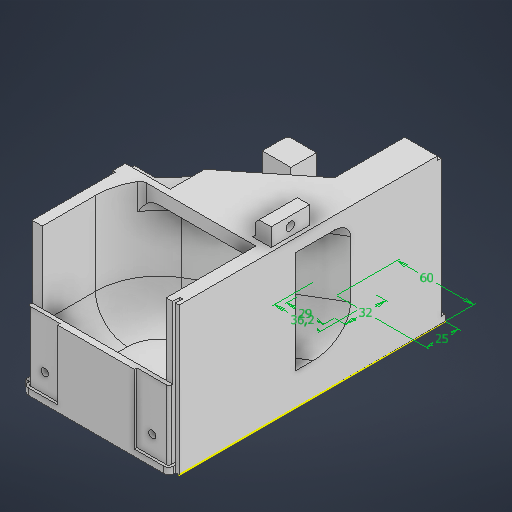
# Autodesk Inventor part: Rampe_V2
Saved by Autodesk Inventor 2026.1 (Build 301233020, 233B)
## iProperties
Created: 2025-05-14
Part Number: Rampe_V2
Material: Generisch
Document SubType Name: Modeling
Designer: iopeter
Density: 1 g/cm^3
Appearance: Vorgabe
Author: iopeter
Autodesk Inventor part; units mm, degrees
ref_plane "YZ Plane" through (0, 0, 0) normal (1, 0, 0) x (0, 1, 0)
ref_plane "XZ Plane" through (0, 0, 0) normal (0, 1, 0) x (-1, 0, 0)
ref_plane "XY Plane" through (0, 0, 0) normal (0, 0, 1) x (1, 0, 0)
ref_plane "Arbeitsebene1" through (-48.5, 0, 84.5) normal (1, 0, 0) x (0, 0, -1)
sketch "Skizze1" plane through (-48.5, 0, 84.5) normal (1, 0, 0) x (0, 0, -1)
  line L0 (81.5, 430) -> (81.5, -250) construction
  line L1 (-117.5, 430) -> (81.5, 430) construction
  line L2 (-117.5, -250) -> (-117.5, 430) construction
  line L3 (81.5, -250) -> (-117.5, -250) construction
  line L4 (81.5, -360) -> (-117.5, -360) construction
  line L5 (-117.5, -360) -> (-117.5, 430) construction
  line L6 (84.5, -360) -> (84.5, 430) construction
  line L7 (84.5, -360) -> (-117.5, -360)
  line L8 (-117.5, -360) -> (-117.5, -250)
  line L9 (-117.5, -250) -> (84.5, -250)
  line L10 (84.5, -250) -> (84.5, -360)
  line L11 (-117.5, -250) -> (-47.5, -250)
  line L12 (-47.5, -250) -> (-47.5, -340)
  line L13 (-47.5, -340) -> (-117.5, -340)
  line L14 (-117.5, -340) -> (-117.5, -250)
  point P0 (84.5, 0)
  point P1 (-117.5, -340)
  dimension "d7" = 70
  dimension "d8" = 90
  constraints: 16 end point, 4 parallel, 2 horizontal, 2 perpendicular, 1 point on line
  measures "d7" distance of L12.end L13.end
  measures "d8" distance of L11.end L12.end
ref_plane "Arbeitsebene2" through (68.5, -430, -3) normal (1, 0, 0) x (0, 1, 0)
extrude "Extrusion1" add sketch "Skizze1" along normal up to surface (117 mm away)
ref_plane "Arbeitsebene4" through (-38.5, 0, 84.5) normal (-1, 0, 0) x (0, 0, 1)
sketch "Skizze4" plane through (-38.5, 0, 84.5) normal (-1, 0, 0) x (0, 0, 1)
  line L0 (47.5, -340) -> (117.5, -340) projected
  line L1 (47.5, -250) -> (47.5, -340) projected
  line L2 (117.5, -250) -> (117.5, -360) projected
  line L3 (-84.5, -360) -> (-84.5, -250) projected
  line L4 (117.5, -360) -> (-84.5, -360) projected
  line L5 (117.5, -250) -> (117.5, -360) projected
  line L6 (-84.5, -250) -> (117.5, -250) projected
  point P0 (-84.5, 0)
extrude "Extrusion4" cut sketch "Skizze4" against normal through all contours L1 L6 L2 L0
sketch "Skizze5" plane through (-38.5, -340, 202) normal (0, 1, 0) x (1, 0, 0)
  line L0 (0, 70) -> (107, 70) projected
  line L1 (107, 70) -> (107, 202) projected
  line L2 (-10, 202) -> (107, 202) projected
  line L3 (-10, 202) -> (-10, 0) projected
  line L4 (-10, 0) -> (0, 0) projected
  line L5 (0, 0) -> (0, 70) projected
  line L6 (0, 70) -> (107, 134)
  point P0 (38.5, 202)
  dimension "d17" = 68
  constraints: 2 end point, 1 point on line
  measures "d17" distance of L1.end L6.end
extrude "Extrusion5" cut sketch "Skizze5" along normal blind 80 contours L6 L1 L0
fillet "Rundung1" radius 50 1 edges at (-38.5, -300, 132)
fillet "Rundung2" radius 25 4 edges at (-31.993, -340, 135.6901) (-38.5, -340, 171.1775) (-38.5, -340, 192) (27.1671, -340, 92.7225)
fillet "Rundung3" radius 10.5 2 edges at (-22.7072, -260, 123.8876) (27.1671, -260, 92.7225)
fillet "Rundung5" radius 3.5 1 edges at (-48.5, -305, 0)
fillet "Rundung8" radius 5 2 edges at (-29.6825, -265.25, 132) (-29.6825, -255, 132)
sketch "Skizze10" plane through (68.5, -340, 202) normal (1, 0, 0) x (0, 0, -1)
  line L0 (70, 90) -> (202, 90) projected
  line L1 (202, 90) -> (202, -20) projected
  line L2 (0, -20) -> (0, 0) projected
  line L3 (0, 0) -> (104.8693, 0) projected
  ellipse E0 centre (104.8693, 25) end of major axis (134, 25) minor radius 25 (104.8693, 0) -> (134, 25) ccw projected
  line L4 (134, 25) -> (134, 69.5) projected
  ellipse E1 centre (121.7651, 69.5) end of major axis (134, 69.5) minor radius 10.5 (134, 69.5) -> (121.7651, 80) ccw projected
  line L5 (121.7651, 80) -> (70, 80) projected
  line L6 (0, 0) -> (71, 0)
  line L7 (71, 0) -> (71, 90)
  line L8 (71, 90) -> (0, 90)
  line L9 (0, 90) -> (0, 0)
  line L10 (70, 80) -> (70, 90) projected
  line L11 (202, -20) -> (0, -20) projected
  point P0 (202, 340)
  point P1 (71, 80)
  constraints: 8 end point, 2 parallel, 1 horizontal, 1 perpendicular, 2 other
extrude "Extrusion9" add sketch "Skizze10" against normal blind 10 contours L10 L5 L7 L3 L9 L8
thicken "Thicken2" operation add thickness 20 both sides no extend neighbours no toward (0, 0, -1) faces at (61.8333, -313.3333, 131)
sketch "Sketch13" plane through (-48.5, -360, 202) normal (0, -1, 0) x (1, 0, 0)
  arc A0 (0, -198.5) -> (3.5, -202) centre (3.5, -198.5) ccw projected
  line L0 (3.5, -202) -> (117, -202) projected
  line L1 (117, -202) -> (117, 0) projected
  line L2 (0, 0) -> (117, 0) projected
  line L3 (0, 0) -> (0, -198.5) projected
  line L4 (-3, -199) -> (0, -199) projected
  line L5 (0, -199) -> (0, 0) projected
  line L6 (-3, 0) -> (0, 0) projected
  line L7 (-3, 0) -> (-3, -199) projected
  line L8 (3, -205) -> (3, -202) projected
  arc A1 (0, -199) -> (3, -202) centre (3, -199) ccw projected
  line L9 (-3, -199) -> (0, -199) projected
  arc A2 (-3, -199) -> (3, -205) centre (3, -199) ccw projected
  line L10 (111, -205) -> (111, -202) projected
  line L11 (111, -202) -> (3, -202) projected
  line L12 (3, -205) -> (3, -202) projected
  line L13 (3, -205) -> (111, -205) projected
  line L14 (117, -202) -> (111, -202)
  line L15 (111, -202) -> (111, -205)
  line L16 (111, -205) -> (117, -205)
  line L17 (117, -205) -> (117, -202)
  point P0 (48.5, -202)
  constraints: 8 end point, 2 parallel, 1 horizontal, 1 perpendicular
extrude "Extrusion11" add sketch "Sketch13" along normal blind 5
fillet "Fillet10" radius 2 1 edges at (68.5, -362.5, -3)
sketch "Sketch14" plane through (-48.5, -365, 202) normal (0, -1, 0) x (1, 0, 0)
  line L0 (27, 5) -> (4, 5) projected
  arc A0 (4, 5) -> (0, 1) centre (4, 1) ccw projected
  line L1 (0, 1) -> (0, -65) projected
  line L2 (110, 5) -> (87, 5) projected
  arc A1 (114, 1) -> (110, 5) centre (110, 1) ccw projected
  line L3 (114, -65) -> (114, 1) projected
  line L4 (27, 5) -> (87, 5)
  line L5 (0, 0) -> (10, 0) projected
  line L6 (0, 0) -> (114, 0)
  point P0 (48.5, -202)
  constraints: 4 end point, 1 collinear, 1 perpendicular, 1 point on line
ref_plane "Work Plane5" through (38.5, -360, 205) normal (0, -1, 0) x (1, 0, 0)
extrude "Extrusion12" add sketch "Sketch14" against normal up to surface (5 mm away)
sketch "Sketch15" plane through (-48.5, -360, 202) normal (0, 1, 0) x (1, 0, 0)
  line L0 (4, -3) -> (27, -3)
  arc A0 (2, -1) -> (4, -3) centre (4, -1) ccw
  line L1 (2, 65) -> (2, -1)
  line L2 (87, -3) -> (110, -3)
  arc A1 (110, -3) -> (112, -1) centre (110, -1) ccw
  line L3 (112, -1) -> (112, 65)
  line L4 (27, -3) -> (87, -3)
  line L5 (107, 0) -> (35, 0)
  line L6 (2, -1) -> (2, 0)
  line L7 (2, 0) -> (112, 0)
  line L8 (112, 0) -> (112, -1)
  arc A2 (110, -3) -> (112, -1) centre (110, -1) ccw
  line L9 (110, -3) -> (87, -3)
  line L10 (87, -3) -> (87, -5)
  line L11 (87, -5) -> (27, -5)
  line L12 (27, -3) -> (27, -5)
  line L13 (27, -3) -> (4, -3)
  arc A3 (2, -1) -> (4, -3) centre (4, -1) ccw
  point P0 (48.5, 202)
extrude "Extrusion13" add sketch "Sketch15" along normal blind 54 contours A0 L1 L7 L5 L3 A1 L2 L4 L0
sketch "Sketch16" plane through (-44.5, -360, 205) normal (0, 0, 1) x (1, 0, 0)
  line L0 (0, 790) -> (0, 0) projected
  line L1 (23, 0) -> (0, 0) projected
  line L2 (23, 117) -> (23, 0) projected
  line L3 (27.5, 117) -> (23, 117) projected
  line L4 (27.5, 674) -> (27.5, 117) projected
  line L5 (23, 674) -> (27.5, 674) projected
  line L6 (23, 790) -> (23, 674) projected
  line L7 (0, 790) -> (23, 790) projected
  line L8 (106, 0) -> (106, 790) projected
  line L9 (83, 790) -> (106, 790) projected
  line L10 (83, 674) -> (83, 790) projected
  line L11 (78.5, 674) -> (83, 674) projected
  line L12 (78.5, 117) -> (78.5, 674) projected
  line L13 (83, 117) -> (78.5, 117) projected
  line L14 (83, 0) -> (83, 117) projected
  line L15 (106, 0) -> (83, 0) projected
  line L16 (106, 0) -> (0, 0) projected
  line L17 (106, 0) -> (106, 54) projected
  line L18 (0, 54) -> (106, 54) projected
  line L19 (0, 0) -> (0, 54) projected
  point P0 (44.5, 360)
  point P1 (83, 54)
  point P2 (23, 54)
ref_plane "Work Plane6" through (-44.5, -360, 207) normal (0, 0, 1) x (1, 0, 0)
extrude "Extrusion14" add sketch "Sketch16" along normal up to surface (2 mm away) contours L18 L14 L16 L2
sketch "Sketch17" plane through (-48.5, -360, 202) normal (0, 1, 0) x (1, 0, 0)
  line L0 (111, 205) -> (111, 202) construction
  arc A0 (117, 203) -> (115, 205) centre (115, 203) ccw construction
  line L1 (3, 205) -> (115, 205) construction
  arc A1 (3, 205) -> (-3, 199) centre (3, 199) ccw projected
  line L2 (-3, 0) -> (-3, 199) projected
  line L3 (0, 0) -> (-3, 0) projected
  line L4 (0, 0) -> (0, 198.5) projected
  arc A2 (3.5, 202) -> (0, 198.5) centre (3.5, 198.5) ccw projected
  line L5 (3.5, 202) -> (117, 202) construction
  line L6 (117, 203) -> (117, 202) construction
  line L7 (111, 202) -> (117, 202)
  line L8 (117, 202) -> (117, 205)
  line L9 (117, 205) -> (111, 205)
  line L10 (111, 205) -> (111, 202)
  point P0 (48.5, 202)
  constraints: 8 end point, 2 parallel, 1 horizontal, 1 perpendicular, 1 other
extrude "Extrusion15" add sketch "Sketch17" along normal blind 107 and the other way blind 5
sketch "Sketch18" plane through (-48.5, -365, 202) normal (0, -1, 0) x (1, 0, 0)
  line L0 (3, -208) -> (117, -208) projected
  line L1 (117, -205) -> (117, -208) projected
  line L2 (117, -205) -> (3, -205) projected
  line L3 (3, -205) -> (3, -208) projected
  point P0 (48.5, -202)
ref_plane "Work Plane7" through (-45.5, -360, -6) normal (0, -1, 0) x (1, 0, 0)
extrude "Extrusion16" add sketch "Sketch18" against normal up to surface (5 mm away)
sketch "Sketch19" plane through (-48.5, 0, 84.5) normal (-1, 0, 0) x (0, 0, 1)
  line L0 (48.5, 430) -> (48.5, -360) projected
  circle A0 centre (108.5, 160) radius 2.5 projected
  circle A1 centre (108.5, -135) radius 2.5 projected
  line L1 (52.5, 430) -> (52.5, -360) projected
  line L2 (118.5, -360) -> (52.5, -360) projected
  line L3 (118.5, 430) -> (118.5, -360) projected
  line L4 (52.5, 430) -> (118.5, 430) projected
  line L5 (48.5, -360) -> (118.5, -360)
  line L6 (118.5, -360) -> (118.5, -250)
  line L7 (118.5, -250) -> (48.5, -250)
  line L8 (48.5, -250) -> (48.5, -360)
  point P0 (-84.5, 0)
  point P1 (117.5, -250)
  point P2 (48.5, -250)
  point P3 (52.5, -250)
  constraints: 8 end point, 2 parallel, 1 horizontal, 1 horizontal alignment, 1 perpendicular, 1 point on line
extrude "Extrusion17" cut sketch "Sketch19" against normal blind 2 contours L7 L3 L2 L1
sketch "Sketch21" plane through (68.5, -250, 202) normal (0, 1, 0) x (1, 0, 0)
  line L0 (0, 0) -> (0, 202) projected
  line L1 (0, 75) -> (-15, 75)
  line L2 (-15, 75) -> (-15, 105)
  line L3 (-15, 105) -> (0, 105)
  line L4 (0, 105) -> (0, 75)
  line L5 (0, 75) -> (-3, 75)
  line L6 (-3, 75) -> (-3, 105)
  line L7 (-3, 105) -> (0, 105)
  line L8 (0, 105) -> (0, 75)
  point P0 (-68.5, 202)
  point P1 (0, 105)
  point P2 (-3, 75)
  dimension "d131" = 15
  dimension "d132" = 30
  dimension "d133" = 75
  dimension "d143" = 3
  constraints: 16 end point, 4 parallel, 2 horizontal, 2 perpendicular, 2 point on line
  measures "d131" distance of L2.end L3.end
  measures "d132" distance of L1.end L2.end
  measures "d133" distance of L0.start L1.start
  measures "d143" distance of L6.end L7.end
extrude "Extrusion19" add sketch "Sketch21" along normal blind 14 contours L1 L2 L3 L6
sketch "Sketch22" plane through (-38.5, -250, 202) normal (0, 1, 0) x (1, 0, 0)
  line L0 (102, 5) -> (104, 5) projected
  line L1 (104, 5) -> (104, -1) projected
  line L2 (102, -1) -> (104, -1) projected
  line L3 (102, -1) -> (102, 5) projected
  line L4 (102, -1) -> (104, -1) projected
  arc A0 (100, -5) -> (104, -1) centre (100, -1) ccw projected
  line L5 (100, -3) -> (100, -5) projected
  arc A1 (100, -3) -> (102, -1) centre (100, -1) ccw projected
  point P0 (38.5, 202)
extrude "Extrusion20" cut sketch "Sketch22" against normal up to surface (110 mm away) contours L0 L1 L2 L3
thicken "Thicken3" operation cut thickness 0.5 both sides no extend neighbours no toward (0, 0, -1) faces at (64.8333, -323.3333, 197)
sketch "Sketch24" plane through (65.5, -250, 127) normal (1, 0, 0) x (0, 0, -1)
  line L0 (30, 0) -> (0, 0) projected
  line L1 (30, 0) -> (30, 14) projected
  line L2 (0, 14) -> (30, 14) projected
  line L3 (0, 0) -> (0, 14) projected
  circle A0 centre (15, 7) radius 3.2
  point P0 (127, 250)
  point P1 (0, 7)
  point P2 (15, 14)
  dimension "d144" = 6.4
  constraints: 2 midpoint, 1 centre point, 1 horizontal alignment, 1 vertical alignment
  measures "d144" diameter of A0
extrude "Extrusion22" cut sketch "Sketch24" against normal through all contours A0
chamfer "Chamfer15" distance 2.5 angle 45 1 edges at (53.5, -250, 112)
chamfer "Chamfer16" distance 2.5 angle 45 1 edges at (53.5, -236, 112)
sketch "Sketch25" plane through (-44.5, -360, 205) normal (0, 0, 1) x (1, 0, 0)
  circle A0 centre (11, 775) radius 2.8 projected
  circle A1 centre (95, 775) radius 2.8 projected
  circle A2 centre (95, 15) radius 2.8
  circle A3 centre (11, 15) radius 2.8
  line L0 (23, 0) -> (0, 0) projected
  point P0 (44.5, 360)
  dimension "d153" = 15
  constraints: 2 centre point, 2 equal radius, 2 vertical alignment, 1 horizontal alignment
  measures "d153" distance from line of L0 A3.centre
extrude "Extrusion23" cut sketch "Sketch25" against normal blind 12 contours A2 | A3
sketch "Skizze26" plane through (-48.5, 0, 84.5) normal (-1, 0, 0) x (0, 0, 1)
  line L0 (12.5, -250) -> (42.5, -250) projected
  line L1 (42.5, -250) -> (-70.5, -250)
  line L2 (-70.5, -250) -> (-70.5, -255)
  line L3 (-70.5, -255) -> (42.5, -255)
  line L4 (42.5, -255) -> (42.5, -250)
  circle A0 centre (18.5, -229.9838) radius 11 projected
  circle A1 centre (-46.5, -229.9838) radius 11 projected
  point P0 (-84.5, 0)
  dimension "d156" = 5
  dimension "d157" = 24
  constraints: 8 end point, 2 parallel, 1 horizontal, 1 perpendicular
  measures "d156" distance between parallel lines of L3 L1
  measures "d157" distance from line of L2 A1.centre
extrude "Extrusion24" cut sketch "Skizze26" against normal blind 35 contours L0 L4 L3 L2 L1
sketch "Skizze27" plane through (-48.5, -365, 202) normal (0, -1, 0) x (1, 0, 0)
  line L0 (42.5, -199) -> (71.5, -199)
  line L1 (71.5, -199) -> (71.5, -167)
  line L2 (71.5, -167) -> (42.5, -167)
  line L3 (42.5, -167) -> (42.5, -199)
  line L4 (42.5, -199) -> (71.5, -167) construction
  line L5 (71.5, -199) -> (42.5, -167) construction
  line L6 (38.9, -183) -> (75.1, -183) construction
  line L7 (117, -208) -> (117, 0) projected
  line L8 (3, -208) -> (117, -208) projected
  point P0 (48.5, -202)
  point P1 (57, -183)
  point P2 (57, -183)
  dimension "d162" = 29
  dimension "d163" = 32
  dimension "d164" = 36.2
  dimension "d165" = 60
  dimension "d166" = 25
  constraints: 14 end point, 3 midpoint, 2 coincident, 2 horizontal, 2 parallel, 1 perpendicular
  measures "d162" distance of L2.end L1.end
  measures "d163" distance of L1.end L0.end
  measures "d164" distance of L6.end L6.start
  measures "d165" distance from line of point (57, -183) L7
  measures "d166" distance from line of L8 point (57, -183)
extrude "Extrusion25" cut sketch "Skizze27" against normal blind 120.75
hole "Bohrung3" at (-9.6, -365, 19) at (26.6, -365, 19) direction (0, 1, 0) diameter 3.3 end through all
thicken "Thicken4" operation cut thickness 0.1 both sides no extend neighbours no toward (1, 0, 0) faces at (65.5, -286.6667, 200.1667)
sketch "Sketch28" plane through (68.5, -250, 202) normal (0, 1, 0) x (1, 0, 0)
  line L0 (-113.5, 202) -> (-6, 202) projected
  line L1 (-25.5, 202) -> (-94.5, 202)
  line L2 (-94.5, 202) -> (-94.5, 147)
  line L3 (-94.5, 147) -> (-25.5, 147)
  line L4 (-25.5, 147) -> (-25.5, 202)
  line L5 (-45.5, 199) -> (-45.5, 167) projected
  line L6 (-74.5, 167) -> (-74.5, 199) projected
  line L7 (-45.5, 167) -> (-74.5, 167) projected
  point P0 (-68.5, 202)
  dimension "d178" = 20
  dimension "d179" = 20
  dimension "d180" = 20
  constraints: 8 end point, 2 parallel, 1 horizontal, 1 perpendicular, 1 point on line
  measures "d178" distance between parallel lines of L4 L5
  measures "d179" distance between parallel lines of L6 L2
  measures "d180" distance between parallel lines of L7 L3
extrude "Extrusion26" cut sketch "Sketch28" against normal blind 100
sketch "Sketch29" plane through (-45, -360, 0) normal (0, 0, -1) x (-1, 0, 0)
  circle A0 centre (-101.5, 55.0162) radius 3 construction
  circle A1 centre (-11.5, 55.0162) radius 3 construction
  circle A2 centre (-101.5, 55.0162) radius 3.2
  circle A3 centre (-11.5, 55.0162) radius 3.2
  point P0 (-45, 360)
  dimension "d183" = 6.4
  dimension "d184" = 6.4
  constraints: 4 coincident, 2 centre point
  measures "d183" diameter of A2
  measures "d184" diameter of A3
extrude "Extrusion27" cut sketch "Sketch29" against normal blind 15
sketch "Skizze30" plane through (68.5, -250, 202) normal (0, 1, 0) x (1, 0, 0)
  line L0 (0, 134) -> (-82.6658, 84.555) projected
  line L1 (-82, 75) -> (-82, 147) projected
  line L2 (-117, 202) -> (-82, 202)
  line L3 (-82, 202) -> (-82, 102)
  line L4 (-82, 102) -> (-117, 102)
  line L5 (-117, 102) -> (-117, 202)
  line L6 (-25.5, 147) -> (-82, 147) projected
  line L7 (-82, 102) -> (-25.5, 147)
  point P0 (-68.5, 202)
  point P1 (-113.5, 202)
  point P2 (-117, 198.5)
  dimension "d187" = 100
  constraints: 10 end point, 2 parallel, 1 horizontal, 1 horizontal alignment, 1 perpendicular, 1 point on line, 1 vertical alignment
  measures "d187" distance of L2.end L3.end
extrude "Extrusion28" cut sketch "Skizze30" against normal blind 45
sketch "Skizze31" plane through (68.5, -295, 202) normal (0, 1, 0) x (1, 0, 0)
  line L0 (-94.5, 147) -> (-25.5, 147) projected
  line L1 (-94.5, 202) -> (-94.5, 147) projected
  line L2 (-113.5, 202) -> (-94.5, 202) projected
  arc A0 (-113.5, 202) -> (-117, 198.5) centre (-113.5, 198.5) ccw projected
  line L3 (-117, 102) -> (-117, 198.5) projected
  line L4 (-82, 102) -> (-117, 102) projected
  line L5 (-25.5, 147) -> (-82, 102) projected
  line L6 (-94.5, 202) -> (-117, 202)
  line L7 (-117, 202) -> (-117, 182)
  line L8 (-117, 182) -> (-94.5, 182)
  line L9 (-94.5, 182) -> (-94.5, 202)
  arc A1 (-82.6658, 84.555) -> (-107, 41.6451) centre (-57, 41.6451) ccw projected
  line L10 (-117, 102) -> (-101, 102)
  line L11 (-101, 102) -> (-101, 82)
  line L12 (-101, 82) -> (-117, 82)
  line L13 (-117, 82) -> (-117, 102)
  line L14 (-82, 102) -> (-101, 82)
  point P0 (-68.5, 202)
  dimension "d190" = 20
  dimension "d193" = 16
  dimension "d194" = 20
  constraints: 18 end point, 4 parallel, 2 horizontal, 2 perpendicular, 1 point on line
  measures "d190" distance of L7.end L6.end
  measures "d193" distance of L11.end L12.end
  measures "d194" distance of L10.end L11.end
extrude "Extrusion29" cut sketch "Skizze31" against normal blind 30 contours L0 L5 L4 L3 L8 L1 | L14 L11 L4 | L11 L12 L13 L4
thicken "Verdickung5" operation cut thickness 100 both sides no extend neighbours no toward (0, 1, 0) faces at (-31.5, -295, 106.6667)
chamfer "Fasen17" distance 5 angle 45 1 edges at (-37.25, -325, 20)
